Autodesk Fusion 360 part; units mm, degrees
(part 2 of 2)
sketch "Sketch1" plane through (0, 0, 0) normal (0, 0, 1) x (1, 0, 0) in component "Component"
  spline S0 degree 5 poles (13.995984, -1.682277) (13.996145, -1.682295) (13.99649, -1.682333) (13.997074, -1.682393) (13.997986, -1.682484) (13.999345, -1.682614) (14.000924, -1.682758) (14.002718, -1.682916) (14.004722, -1.683085) (14.006931, -1.683262) (14.009338, -1.683445) (14.011941, -1.683633) (14.014736, -1.683823) (14.01772, -1.684015) (14.020889, -1.684207) (14.024241, -1.684397) (14.027771, -1.684584) (14.031477, -1.684766) (14.035355, -1.684942) (14.039402, -1.685111) (14.043617, -1.685272) (14.047995, -1.685422) (14.052535, -1.685562) (14.057234, -1.685689) (14.062089, -1.685804) (14.067098, -1.685904) (14.072259, -1.685988) (14.077569, -1.686056) (14.083026, -1.686107) (14.088629, -1.68614) (14.094374, -1.686154) (14.100261, -1.686147) (14.106286, -1.686119) (14.112449, -1.68607) (14.118747, -1.685998) (14.125178, -1.685903) (14.13174, -1.685783) (14.138433, -1.685639) (14.145254, -1.685469) (14.152202, -1.685272) (14.159274, -1.685049) (14.16647, -1.684797) (14.173787, -1.684518) (14.181225, -1.684209) (14.188782, -1.68387) (14.196456, -1.683501) (14.204247, -1.683101) (14.212151, -1.68267) (14.220169, -1.682207) (14.228299, -1.681711) (14.23654, -1.681182) (14.24489, -1.680619) (14.253348, -1.680022) (14.261913, -1.67939) (14.270584, -1.678723) (14.279359, -1.67802) (14.288238, -1.677281) (14.297218, -1.676505) (14.3063, -1.675692) (14.315482, -1.674842) (14.324762, -1.673954) (14.334141, -1.673027) (14.343616, -1.672061) (14.353187, -1.671056) (14.362853, -1.670012) (14.372612, -1.668927) (14.382464, -1.667802) (14.392408, -1.666636) (14.402443, -1.665429) (14.412568, -1.66418) (14.422782, -1.66289) (14.433084, -1.661557) (14.443473, -1.660182) (14.453948, -1.658763) (14.464509, -1.657302) (14.475155, -1.655797) (14.485884, -1.654247) (14.496696, -1.652654) (14.50759, -1.651016) (14.518565, -1.649334) (14.529621, -1.647606) (14.540757, -1.645833) (14.551972, -1.644014) (14.563264, -1.642149) (14.574634, -1.640238) (14.586081, -1.638281) (14.597604, -1.636276) (14.609202, -1.634225) (14.620874, -1.632127) (14.63262, -1.629981) (14.644439, -1.627787) (14.65633, -1.625545) (14.668293, -1.623255) (14.680327, -1.620916) (14.692431, -1.618529) (14.704605, -1.616093) (14.716848, -1.613607) (14.729159, -1.611073) (14.741538, -1.608488) (14.753984, -1.605854) (14.766497, -1.60317) (14.779075, -1.600436) (14.791718, -1.597652) (14.804426, -1.594816) (14.817198, -1.59193) (14.830033, -1.588994) (14.842931, -1.586006) (14.855891, -1.582966) (14.868913, -1.579875) (14.881995, -1.576733) (14.895139, -1.573538) (14.908342, -1.570292) (14.921604, -1.566993) (14.934926, -1.563642) (14.948305, -1.560239) (14.961743, -1.556783) (14.975237, -1.553274) (14.988788, -1.549712) (15.002395, -1.546097) (15.016058, -1.542429) (15.029776, -1.538707) (15.043548, -1.534932) (15.057375, -1.531103) (15.071255, -1.52722) (15.085188, -1.523283) (15.099173, -1.519292) (15.113211, -1.515247) (15.1273, -1.511148) (15.14144, -1.506993) (15.155631, -1.502785) (15.169872, -1.498521) (15.184163, -1.494203) (15.198502, -1.48983) (15.212891, -1.485402) (15.227328, -1.480918) (15.241812, -1.476379) (15.256344, -1.471785) (15.270923, -1.467135) (15.285548, -1.46243) (15.30022, -1.457669) (15.314936, -1.452852) (15.329698, -1.447979) (15.344505, -1.44305) (15.359356, -1.438064) (15.374251, -1.433023) (15.389189, -1.427925) (15.40417, -1.422771) (15.419194, -1.41756) (15.43426, -1.412293) (15.449368, -1.406969) (15.464517, -1.401588) (15.479707, -1.39615) (15.494937, -1.390656) (15.510208, -1.385104) (15.525518, -1.379495) (15.540868, -1.373829) (15.556256, -1.368106) (15.571683, -1.362325) (15.587148, -1.356487) (15.602651, -1.350592) (15.618192, -1.344639) (15.633769, -1.338628) (15.649383, -1.33256) (15.665034, -1.326434) (15.68072, -1.32025) (15.696441, -1.314008) (15.712198, -1.307708) (15.72799, -1.301351) (15.743816, -1.294935) (15.759676, -1.288461) (15.77557, -1.281929) (15.791497, -1.275338) (15.807457, -1.26869) (15.823449, -1.261983) (15.839474, -1.255217) (15.855531, -1.248393) (15.871619, -1.241511) (15.887739, -1.23457) (15.903889, -1.22757) (15.92007, -1.220512) (15.936281, -1.213395) (15.952522, -1.206219) (15.968793, -1.198985) (15.985093, -1.191692) (16.001421, -1.184339) (16.017778, -1.176928) (16.034164, -1.169458) (16.050577, -1.161929) (16.067018, -1.154341) (16.083486, -1.146694) (16.09998, -1.138988) (16.116502, -1.131222) (16.13305, -1.123398) (16.149623, -1.115514) (16.166222, -1.107571) (16.182847, -1.099569) (16.199497, -1.091508) (16.216171, -1.083387) (16.232869, -1.075206) (16.249592, -1.066967) (16.266339, -1.058668) (16.283109, -1.05031) (16.299902, -1.041892) (16.316718, -1.033414) (16.333556, -1.024878) (16.350417, -1.016281) (16.3673, -1.007625) (16.384205, -0.99891) (16.401131, -0.990135) (16.418077, -0.9813) (16.435045, -0.972406) (16.452034, -0.963452) (16.469042, -0.954438) (16.48607, -0.945365) (16.503119, -0.936232) (16.520186, -0.92704) (16.537273, -0.917787) (16.554378, -0.908475) (16.571502, -0.899104) (16.588644, -0.889672) (16.605804, -0.880181) (16.622982, -0.87063) (16.640177, -0.861019) (16.65739, -0.851349) (16.674619, -0.841618) (16.691864, -0.831828) (16.709127, -0.821978) (16.726405, -0.812068) (16.743699, -0.802099) (16.761008, -0.79207) (16.778333, -0.78198) (16.795673, -0.771831) (16.813028, -0.761623) (16.830397, -0.751354) (16.84778, -0.741025) (16.865177, -0.730637) (16.882588, -0.720189) (16.900012, -0.709681) (16.917449, -0.699113) (16.934898, -0.688486) (16.952361, -0.677798) (16.966342, -0.669201) (16.976834, -0.662726) (16.98383, -0.658397) (16.987329, -0.656229) knots 0 0 0 0 0 0 0.00416667 0.00833333 0.0125 0.01666667 0.02083333 0.025 0.02916667 0.03333333 0.0375 0.04166667 0.04583333 0.05 0.05416667 0.05833333 0.0625 0.06666667 0.07083333 0.075 0.07916667 0.08333333 0.0875 0.09166667 0.09583333 0.1 0.10416667 0.10833333 0.1125 0.11666667 0.12083333 0.125 0.12916667 0.13333333 0.1375 0.14166667 0.14583333 0.15 0.15416667 0.15833333 0.1625 0.16666667 0.17083333 0.175 0.17916667 0.18333333 0.1875 0.19166667 0.19583333 0.2 0.20416667 0.20833333 0.2125 0.21666667 0.22083333 0.225 0.22916667 0.23333333 0.2375 0.24166667 0.24583333 0.25 0.25416667 0.25833333 0.2625 0.26666667 0.27083333 0.275 0.27916667 0.28333333 0.2875 0.29166667 0.29583333 0.3 0.30416667 0.30833333 0.3125 0.31666667 0.32083333 0.325 0.32916667 0.33333333 0.3375 0.34166667 0.34583333 0.35 0.35416667 0.35833333 0.3625 0.36666667 0.37083333 0.375 0.37916667 0.38333333 0.3875 0.39166667 0.39583333 0.4 0.40416667 0.40833333 0.4125 0.41666667 0.42083333 0.425 0.42916667 0.43333333 0.4375 0.44166667 0.44583333 0.45 0.45416667 0.45833333 0.4625 0.46666667 0.47083333 0.475 0.47916667 0.48333333 0.4875 0.49166667 0.49583333 0.5 0.50416667 0.50833333 0.5125 0.51666667 0.52083333 0.525 0.52916667 0.53333333 0.5375 0.54166667 0.54583333 0.55 0.55416667 0.55833333 0.5625 0.56666667 0.57083333 0.575 0.57916667 0.58333333 0.5875 0.59166667 0.59583333 0.6 0.60416667 0.60833333 0.6125 0.61666667 0.62083333 0.625 0.62916667 0.63333333 0.6375 0.64166667 0.64583333 0.65 0.65416667 0.65833333 0.6625 0.66666667 0.67083333 0.675 0.67916667 0.68333333 0.6875 0.69166667 0.69583333 0.7 0.70416667 0.70833333 0.7125 0.71666667 0.72083333 0.725 0.72916667 0.73333333 0.7375 0.74166667 0.74583333 0.75 0.75416667 0.75833333 0.7625 0.76666667 0.77083333 0.775 0.77916667 0.78333333 0.7875 0.79166667 0.79583333 0.8 0.80416667 0.80833333 0.8125 0.81666667 0.82083333 0.825 0.82916667 0.83333333 0.8375 0.84166667 0.84583333 0.85 0.85416667 0.85833333 0.8625 0.86666667 0.87083333 0.875 0.87916667 0.88333333 0.8875 0.89166667 0.89583333 0.9 0.90416667 0.90833333 0.9125 0.91666667 0.92083333 0.925 0.92916667 0.93333333 0.9375 0.94166667 0.94583333 0.95 0.95416667 0.95833333 0.9625 0.96666667 0.97083333 0.975 0.97916667 0.98333333 0.9875 0.99166667 0.99583333 1 1 1 1 1 1
  spline S1 degree 5 poles (13.995984, 1.682277) (13.996145, 1.682295) (13.99649, 1.682333) (13.997074, 1.682393) (13.997986, 1.682484) (13.999345, 1.682614) (14.000924, 1.682758) (14.002718, 1.682916) (14.004722, 1.683085) (14.006931, 1.683262) (14.009338, 1.683445) (14.011941, 1.683633) (14.014736, 1.683823) (14.01772, 1.684015) (14.020889, 1.684207) (14.024241, 1.684397) (14.027771, 1.684584) (14.031477, 1.684766) (14.035355, 1.684942) (14.039402, 1.685111) (14.043617, 1.685272) (14.047995, 1.685422) (14.052535, 1.685562) (14.057234, 1.685689) (14.062089, 1.685804) (14.067098, 1.685904) (14.072259, 1.685988) (14.077569, 1.686056) (14.083026, 1.686107) (14.088629, 1.68614) (14.094374, 1.686154) (14.100261, 1.686147) (14.106286, 1.686119) (14.112449, 1.68607) (14.118747, 1.685998) (14.125178, 1.685903) (14.13174, 1.685783) (14.138433, 1.685639) (14.145254, 1.685469) (14.152202, 1.685272) (14.159274, 1.685049) (14.16647, 1.684797) (14.173787, 1.684518) (14.181225, 1.684209) (14.188782, 1.68387) (14.196456, 1.683501) (14.204247, 1.683101) (14.212151, 1.68267) (14.220169, 1.682207) (14.228299, 1.681711) (14.23654, 1.681182) (14.24489, 1.680619) (14.253348, 1.680022) (14.261913, 1.67939) (14.270584, 1.678723) (14.279359, 1.67802) (14.288238, 1.677281) (14.297218, 1.676505) (14.3063, 1.675692) (14.315482, 1.674842) (14.324762, 1.673954) (14.334141, 1.673027) (14.343616, 1.672061) (14.353187, 1.671056) (14.362853, 1.670012) (14.372612, 1.668927) (14.382464, 1.667802) (14.392408, 1.666636) (14.402443, 1.665429) (14.412568, 1.66418) (14.422782, 1.66289) (14.433084, 1.661557) (14.443473, 1.660182) (14.453948, 1.658763) (14.464509, 1.657302) (14.475155, 1.655797) (14.485884, 1.654247) (14.496696, 1.652654) (14.50759, 1.651016) (14.518565, 1.649334) (14.529621, 1.647606) (14.540757, 1.645833) (14.551972, 1.644014) (14.563264, 1.642149) (14.574634, 1.640238) (14.586081, 1.638281) (14.597604, 1.636276) (14.609202, 1.634225) (14.620874, 1.632127) (14.63262, 1.629981) (14.644439, 1.627787) (14.65633, 1.625545) (14.668293, 1.623255) (14.680327, 1.620916) (14.692431, 1.618529) (14.704605, 1.616093) (14.716848, 1.613607) (14.729159, 1.611073) (14.741538, 1.608488) (14.753984, 1.605854) (14.766497, 1.60317) (14.779075, 1.600436) (14.791718, 1.597652) (14.804426, 1.594816) (14.817198, 1.59193) (14.830033, 1.588994) (14.842931, 1.586006) (14.855891, 1.582966) (14.868913, 1.579875) (14.881995, 1.576733) (14.895139, 1.573538) (14.908342, 1.570292) (14.921604, 1.566993) (14.934926, 1.563642) (14.948305, 1.560239) (14.961743, 1.556783) (14.975237, 1.553274) (14.988788, 1.549712) (15.002395, 1.546097) (15.016058, 1.542429) (15.029776, 1.538707) (15.043548, 1.534932) (15.057375, 1.531103) (15.071255, 1.52722) (15.085188, 1.523283) (15.099173, 1.519292) (15.113211, 1.515247) (15.1273, 1.511148) (15.14144, 1.506993) (15.155631, 1.502785) (15.169872, 1.498521) (15.184163, 1.494203) (15.198502, 1.48983) (15.212891, 1.485402) (15.227328, 1.480918) (15.241812, 1.476379) (15.256344, 1.471785) (15.270923, 1.467135) (15.285548, 1.46243) (15.30022, 1.457669) (15.314936, 1.452852) (15.329698, 1.447979) (15.344505, 1.44305) (15.359356, 1.438064) (15.374251, 1.433023) (15.389189, 1.427925) (15.40417, 1.422771) (15.419194, 1.41756) (15.43426, 1.412293) (15.449368, 1.406969) (15.464517, 1.401588) (15.479707, 1.39615) (15.494937, 1.390656) (15.510208, 1.385104) (15.525518, 1.379495) (15.540868, 1.373829) (15.556256, 1.368106) (15.571683, 1.362325) (15.587148, 1.356487) (15.602651, 1.350592) (15.618192, 1.344639) (15.633769, 1.338628) (15.649383, 1.33256) (15.665034, 1.326434) (15.68072, 1.32025) (15.696441, 1.314008) (15.712198, 1.307708) (15.72799, 1.301351) (15.743816, 1.294935) (15.759676, 1.288461) (15.77557, 1.281929) (15.791497, 1.275338) (15.807457, 1.26869) (15.823449, 1.261983) (15.839474, 1.255217) (15.855531, 1.248393) (15.871619, 1.241511) (15.887739, 1.23457) (15.903889, 1.22757) (15.92007, 1.220512) (15.936281, 1.213395) (15.952522, 1.206219) (15.968793, 1.198985) (15.985093, 1.191692) (16.001421, 1.184339) (16.017778, 1.176928) (16.034164, 1.169458) (16.050577, 1.161929) (16.067018, 1.154341) (16.083486, 1.146694) (16.09998, 1.138988) (16.116502, 1.131222) (16.13305, 1.123398) (16.149623, 1.115514) (16.166222, 1.107571) (16.182847, 1.099569) (16.199497, 1.091508) (16.216171, 1.083387) (16.232869, 1.075206) (16.249592, 1.066967) (16.266339, 1.058668) (16.283109, 1.05031) (16.299902, 1.041892) (16.316718, 1.033414) (16.333556, 1.024878) (16.350417, 1.016281) (16.3673, 1.007625) (16.384205, 0.99891) (16.401131, 0.990135) (16.418077, 0.9813) (16.435045, 0.972406) (16.452034, 0.963452) (16.469042, 0.954438) (16.48607, 0.945365) (16.503119, 0.936232) (16.520186, 0.92704) (16.537273, 0.917787) (16.554378, 0.908475) (16.571502, 0.899104) (16.588644, 0.889672) (16.605804, 0.880181) (16.622982, 0.87063) (16.640177, 0.861019) (16.65739, 0.851349) (16.674619, 0.841618) (16.691864, 0.831828) (16.709127, 0.821978) (16.726405, 0.812068) (16.743699, 0.802099) (16.761008, 0.79207) (16.778333, 0.78198) (16.795673, 0.771831) (16.813028, 0.761623) (16.830397, 0.751354) (16.84778, 0.741025) (16.865177, 0.730637) (16.882588, 0.720189) (16.900012, 0.709681) (16.917449, 0.699113) (16.934898, 0.688486) (16.952361, 0.677798) (16.966342, 0.669201) (16.976834, 0.662726) (16.98383, 0.658397) (16.987329, 0.656229) knots 0 0 0 0 0 0 0.00416667 0.00833333 0.0125 0.01666667 0.02083333 0.025 0.02916667 0.03333333 0.0375 0.04166667 0.04583333 0.05 0.05416667 0.05833333 0.0625 0.06666667 0.07083333 0.075 0.07916667 0.08333333 0.0875 0.09166667 0.09583333 0.1 0.10416667 0.10833333 0.1125 0.11666667 0.12083333 0.125 0.12916667 0.13333333 0.1375 0.14166667 0.14583333 0.15 0.15416667 0.15833333 0.1625 0.16666667 0.17083333 0.175 0.17916667 0.18333333 0.1875 0.19166667 0.19583333 0.2 0.20416667 0.20833333 0.2125 0.21666667 0.22083333 0.225 0.22916667 0.23333333 0.2375 0.24166667 0.24583333 0.25 0.25416667 0.25833333 0.2625 0.26666667 0.27083333 0.275 0.27916667 0.28333333 0.2875 0.29166667 0.29583333 0.3 0.30416667 0.30833333 0.3125 0.31666667 0.32083333 0.325 0.32916667 0.33333333 0.3375 0.34166667 0.34583333 0.35 0.35416667 0.35833333 0.3625 0.36666667 0.37083333 0.375 0.37916667 0.38333333 0.3875 0.39166667 0.39583333 0.4 0.40416667 0.40833333 0.4125 0.41666667 0.42083333 0.425 0.42916667 0.43333333 0.4375 0.44166667 0.44583333 0.45 0.45416667 0.45833333 0.4625 0.46666667 0.47083333 0.475 0.47916667 0.48333333 0.4875 0.49166667 0.49583333 0.5 0.50416667 0.50833333 0.5125 0.51666667 0.52083333 0.525 0.52916667 0.53333333 0.5375 0.54166667 0.54583333 0.55 0.55416667 0.55833333 0.5625 0.56666667 0.57083333 0.575 0.57916667 0.58333333 0.5875 0.59166667 0.59583333 0.6 0.60416667 0.60833333 0.6125 0.61666667 0.62083333 0.625 0.62916667 0.63333333 0.6375 0.64166667 0.64583333 0.65 0.65416667 0.65833333 0.6625 0.66666667 0.67083333 0.675 0.67916667 0.68333333 0.6875 0.69166667 0.69583333 0.7 0.70416667 0.70833333 0.7125 0.71666667 0.72083333 0.725 0.72916667 0.73333333 0.7375 0.74166667 0.74583333 0.75 0.75416667 0.75833333 0.7625 0.76666667 0.77083333 0.775 0.77916667 0.78333333 0.7875 0.79166667 0.79583333 0.8 0.80416667 0.80833333 0.8125 0.81666667 0.82083333 0.825 0.82916667 0.83333333 0.8375 0.84166667 0.84583333 0.85 0.85416667 0.85833333 0.8625 0.86666667 0.87083333 0.875 0.87916667 0.88333333 0.8875 0.89166667 0.89583333 0.9 0.90416667 0.90833333 0.9125 0.91666667 0.92083333 0.925 0.92916667 0.93333333 0.9375 0.94166667 0.94583333 0.95 0.95416667 0.95833333 0.9625 0.96666667 0.97083333 0.975 0.97916667 0.98333333 0.9875 0.99166667 0.99583333 1 1 1 1 1 1
  spline S2 degree 5 poles (13.994657, -1.68213) (13.994711, -1.682136) (13.994817, -1.682148) (13.994976, -1.682166) (13.995188, -1.682189) (13.995453, -1.682218) (13.995665, -1.682242) (13.995825, -1.68226) (13.995931, -1.682271) (13.995984, -1.682277) knots 0 0 0 0 0 0 0.2 0.4 0.6 0.8 1 1 1 1 1 1
  spline S3 degree 5 poles (13.994657, 1.68213) (13.994711, 1.682136) (13.994817, 1.682148) (13.994976, 1.682166) (13.995188, 1.682189) (13.995453, 1.682218) (13.995665, 1.682242) (13.995825, 1.68226) (13.995931, 1.682271) (13.995984, 1.682277) knots 0 0 0 0 0 0 0.2 0.4 0.6 0.8 1 1 1 1 1 1
  line L0 (0, 0) -> (13.994657, -1.68213)
  line L1 (0, 0) -> (13.994657, 1.68213)
  arc A0 (16.987329, -0.656229) -> (16.987329, 0.656229) centre (0, 0) ccw
  point P0 (13.999968, -1.68267)
  point P1 (14.006616, -1.683235)
  point P2 (14.015933, -1.683899)
  point P3 (14.027922, -1.684588)
  point P4 (14.042586, -1.68523)
  point P5 (14.059926, -1.68575)
  point P6 (14.079939, -1.686076)
  point P7 (14.102623, -1.686133)
  point P8 (14.127975, -1.685849)
  point P9 (14.155988, -1.68515)
  point P10 (14.186656, -1.683962)
  point P11 (14.21997, -1.682212)
  point P12 (14.255919, -1.679828)
  point P13 (14.294493, -1.676737)
  point P14 (14.335677, -1.672865)
  point P15 (14.379458, -1.668141)
  point P16 (14.425819, -1.662492)
  point P17 (14.474742, -1.655848)
  point P18 (14.526208, -1.648135)
  point P19 (14.580197, -1.639283)
  point P20 (14.636686, -1.629221)
  point P21 (14.695653, -1.617879)
  point P22 (14.757071, -1.605187)
  point P23 (14.820915, -1.591075)
  point P24 (14.887156, -1.575474)
  point P25 (14.955766, -1.558315)
  point P26 (15.026712, -1.539532)
  point P27 (15.099964, -1.519055)
  point P28 (15.175488, -1.496819)
  point P29 (15.253247, -1.472757)
  point P30 (15.333207, -1.446804)
  point P31 (15.415329, -1.418894)
  point P32 (15.499574, -1.388964)
  point P33 (15.585901, -1.356949)
  point P34 (15.674269, -1.322787)
  point P35 (15.764635, -1.286416)
  point P36 (15.856953, -1.247775)
  point P37 (15.951178, -1.206804)
  point P38 (16.047263, -1.163441)
  point P39 (16.14516, -1.11763)
  point P40 (16.244818, -1.069312)
  point P41 (16.346188, -1.01843)
  point P42 (16.449216, -0.964928)
  point P43 (16.553849, -0.908752)
  point P44 (16.660034, -0.849846)
  point P45 (16.767714, -0.788158)
  point P46 (16.876831, -0.723636)
  point P47 (13.999968, 1.68267)
  point P48 (14.006616, 1.683235)
  point P49 (14.015933, 1.683899)
  point P50 (14.027922, 1.684588)
  point P51 (14.042586, 1.68523)
  point P52 (14.059926, 1.68575)
  point P53 (14.079939, 1.686076)
  point P54 (14.102623, 1.686133)
  point P55 (14.127975, 1.685849)
  point P56 (14.155988, 1.68515)
  point P57 (14.186656, 1.683962)
  point P58 (14.21997, 1.682212)
  point P59 (14.255919, 1.679828)
  point P60 (14.294493, 1.676737)
  point P61 (14.335677, 1.672865)
  point P62 (14.379458, 1.668141)
  point P63 (14.425819, 1.662492)
  point P64 (14.474742, 1.655848)
  point P65 (14.526208, 1.648135)
  point P66 (14.580197, 1.639283)
  point P67 (14.636686, 1.629221)
  point P68 (14.695653, 1.617879)
  point P69 (14.757071, 1.605187)
  point P70 (14.820915, 1.591075)
  point P71 (14.887156, 1.575474)
  point P72 (14.955766, 1.558315)
  point P73 (15.026712, 1.539532)
  point P74 (15.099964, 1.519055)
  point P75 (15.175488, 1.496819)
  point P76 (15.253247, 1.472757)
  point P77 (15.333207, 1.446804)
  point P78 (15.415329, 1.418894)
  point P79 (15.499574, 1.388964)
  point P80 (15.585901, 1.356949)
  point P81 (15.674269, 1.322787)
  point P82 (15.764635, 1.286416)
  point P83 (15.856953, 1.247775)
  point P84 (15.951178, 1.206804)
  point P85 (16.047263, 1.163441)
  point P86 (16.14516, 1.11763)
  point P87 (16.244818, 1.069312)
  point P88 (16.346188, 1.01843)
  point P89 (16.449216, 0.964928)
  point P90 (16.553849, 0.908752)
  point P91 (16.660034, 0.849846)
  point P92 (16.767714, 0.788158)
  point P93 (16.876831, 0.723636)
sketch "Sketch2" plane through (0, 0, 0) normal (0, 0, 1) x (1, 0, 0) in component "Component"
  circle A0 centre (0, 0) radius 12.5
extrude "Extrude1" add sketch "Sketch2" along normal blind 6.35 contours A0 picked at (-3.387945, -0.621009) makes body 1 in component "Component"
extrude "Extrude2" add sketch "Sketch1" along normal blind 6.35 separate body contours S0 S1 L0 L1 A0 picked at (9.330656, 0) makes body 2 in component "Component"
pattern_circular "C-Pattern1" count 15 over 360 about axis through (0, 0, 1.75) along (0, 0, 1) of "Extrude2" makes body 3 at (4.49007, 1.385281, 2.116667) makes body 4 at (3.538439, 3.091793, 2.116667) makes body 5 at (0.908352, 4.610275, 2.116667) makes body 6 at (0.070028, 4.698386, 2.116667) makes body 7 at (-2.818296, 3.759913, 2.116667) makes body 8 at (-3.444724, 3.195875, 2.116667) makes body 9 at (-4.446791, 1.518481, 2.116667) makes body 10 at (-4.679968, -0.421471, 2.116667) makes body 11 at (-4.103935, -2.288547, 2.116667) makes body 12 at (-2.818296, -3.759913, 2.116667) makes body 13 at (0.070028, -4.698386, 2.116667) makes body 14 at (1.974979, -4.263706, 2.116667) makes body 15 at (3.538439, -3.091793, 2.116667) makes body 16 at (4.033908, -2.409839, 2.116667) in component "Component"
combine "Combine1" operation add target body 1 tool bodies 2 3 4 5 6 7 8 9 10 11 12 13 14 15 16 in component "Component"
sketch "Sketch3" plane through (0, 0, 0) normal (0, 0, 1) x (1, 0, 0) in component "Component"
  line L0 (0, 0) -> (50.859375, 0) construction
  line L1 (50.859375, 0) -> (50.859375, 3) construction
  line L2 (50.859375, 3) -> (0, 3) construction
  line L3 (0, 3) -> (0, 0) construction
  constraint perpendicular L0 L1
  constraint parallel L0 L2
  constraint parallel L1 L3
ref_plane "WorkPlane1" through (0.130063, 0, 6.35) normal (0, 0, 1) x (1, 0, 0)
sketch "Sketch1 (2)" plane through (0, 0, 6.35) normal (0, 0, 1) x (1, 0, 0)
  circle A0 centre (0, 0) radius 12.5
  circle A1 centre (0, 0) radius 20
  line L0 (0, 0) -> (-20, 0)
  line L1 (0, 0) -> (16.18034, -11.755705)
  point P0 (2.416381, 12.264221)
  dimension "d15" = 40
  dimension "d16" = 216
  constraint coincident A0.centre A1.centre
  constraint coincident A1 L0.end
  constraint horizontal L0
  measures "d15" diameter of A1
extrude "Extrude3" cut sketch "Sketch1 (2)" against normal through all contours A0 A1 L0 L1 picked at (13.124223, -11.507785) bodies 1 in component "Component"
component "Component" placed x (1, 0, 0) y (0, 1, 0) z (0, 0, 1) at (0, 0, 0)
equation "NumTeeth = 9"
equation "d16 = ( 24 * NumTeeth ) * 1 deg"

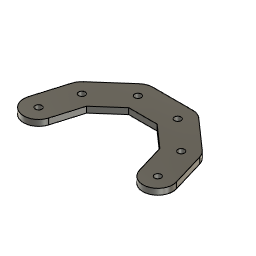
design "GearPlateV2"
Autodesk Fusion 360 part; units mm, degrees
sketch "Sketch1" plane through (0, 0, 0) normal (0, 0, 1) x (1, 0, 0)
  circle A0 centre (0, 0) radius 3.275
  circle A1 centre (120, 0) radius 3.275
  circle A2 centre (120, 0) radius 15 construction
  circle A3 centre (0, 0) radius 15 construction
  circle A4 centre (120, 0) radius 15 construction
  circle A5 centre (10, 33.541) radius 20 construction
  circle A6 centre (40, 59.9985) radius 20 construction
  circle A7 centre (110, 33.541) radius 20 construction
  circle A8 centre (80, 59.9985) radius 20 construction
  circle A9 centre (109.7709, 71.7327) radius 12 construction
  line L0 (143.6237, 88.934) -> (255.6237, 88.934) construction
  circle A10 centre (59.9233, -6.3144) radius 27.5 construction
  circle A11 centre (0, 0) radius 15 construction
  line L1 (150, 0) -> (-15, 0) construction
  circle A12 centre (0, 0) radius 17 construction
  circle A13 centre (120, 0) radius 17 construction
  circle A14 centre (10, 33.541) radius 3.275
  circle A15 centre (40, 59.9985) radius 3.275
  circle A16 centre (80, 59.9985) radius 3.275
  circle A17 centre (110, 33.541) radius 3.275
  circle A18 centre (0, 0) radius 15
  circle A19 centre (10, 33.541) radius 15
  circle A20 centre (40, 59.9985) radius 15
  circle A21 centre (80, 59.9985) radius 15
  circle A22 centre (110, 33.541) radius 15
  circle A23 centre (120, 0) radius 15
  line L2 (-14.3747, 4.2857) -> (-4.3747, 37.8267)
  line L3 (0.0784, 44.791) -> (30.0784, 71.2485)
  line L4 (40, 74.9985) -> (80, 74.9985)
  line L5 (14.3747, -4.2857) -> (24.3747, 29.2553)
  line L6 (19.9216, 22.291) -> (49.9216, 48.7485)
  line L7 (40, 44.9985) -> (80, 44.9985)
  line L8 (70.0784, 48.7485) -> (100.0784, 22.291)
  line L9 (89.9216, 71.2485) -> (119.9216, 44.791)
  line L10 (95.6253, 29.2553) -> (105.6253, -4.2857)
  line L11 (124.3747, 37.8267) -> (134.3747, 4.2857)
  point P0 (105, 0)
  point P1 (15, 0)
  dimension "d2" = 6.55
  dimension "d3" = 6.55
  dimension "d4" = 120
  dimension "d7" = 30
  dimension "d10" = 30
  dimension "d11" = 30
  dimension "d20" = 40
  dimension "d26" = 24
  dimension "d27" = 112
  dimension "d28" = 55
  dimension "d31" = 30
  dimension "d33" = 165
  dimension "d35" = 90
  dimension "d36" = 100
  dimension "d37" = 34
  dimension "d38" = 34
  dimension "d40" = 6.55
  dimension "d41" = 6.55
  dimension "d42" = 6.55
  dimension "d43" = 6.55
  dimension "d44" = 30
  dimension "d45" = 30
  dimension "d46" = 30
  dimension "d47" = 30
  dimension "d48" = 30
  dimension "d49" = 30
  constraint coincident A0.centre A3.centre
  constraint horizontal A0.centre A1.centre
  constraint concentric A1 A2
  constraint concentric A0 A3
  constraint concentric A1 A4
  constraint tangent A3 A5
  constraint tangent A4 A7
  constraint tangent A7 A8
  constraint tangent A6 A8
  constraint tangent A5 A6
  constraint tangent A8 A9
  constraint horizontal L0
  constraint horizontal A6.centre A8.centre
  constraint horizontal A5.centre A7.centre
  constraint concentric A3 A11
  constraint coincident A11 L1.end
  constraint horizontal L1
  constraint coincident A2 P0
  constraint coincident L1 P0
  constraint coincident A11 P1
  constraint coincident L1 P1
  constraint equal A5 A6
  constraint equal A6 A8
  constraint equal A7 A8
  constraint concentric A3 A12
  constraint concentric A4 A13
  constraint concentric A5 A14
  constraint concentric A6 A15
  constraint concentric A8 A16
  constraint concentric A7 A17
  constraint concentric A12 A18
  constraint concentric A14 A19
  constraint concentric A6 A20
  constraint concentric A16 A21
  constraint concentric A17 A22
  constraint concentric A1 A23
  constraint coincident A3 L2.start
  constraint coincident A19 L2.end
  constraint tangent A19 L2
  constraint coincident A19 L3.start
  constraint coincident A20 L3.end
  constraint tangent A20 L3
  constraint coincident A20 L4.start
  constraint coincident A21 L4.end
  constraint tangent A21 L4
  constraint coincident A3 L5.start
  constraint coincident A19 L5.end
  constraint tangent A19 L5
  constraint coincident A19 L6.start
  constraint coincident A20 L6.end
  constraint tangent A20 L6
  constraint coincident A20 L7.start
  constraint coincident A21 L7.end
  constraint tangent A21 L7
  constraint coincident A21 L8.start
  constraint coincident A22 L8.end
  constraint tangent A22 L8
  constraint coincident A21 L9.start
  constraint coincident A22 L9.end
  constraint tangent A22 L9
  constraint coincident A22 L10.start
  constraint coincident A2 L10.end
  constraint tangent A2 L10
  constraint coincident A22 L11.start
  constraint coincident A2 L11.end
  constraint tangent A2 L11
  constraint tangent A22 L11
  constraint tangent A22 L10
  constraint tangent A21 L8
  constraint tangent A21 L9
  constraint tangent A20 L4
  constraint tangent A20 L7
  constraint tangent A19 L6
  constraint tangent A3 L5
  constraint tangent A3 L2
  constraint tangent A19 L3
  measures "d2" diameter of A0
  measures "d3" diameter of A1
  measures "d4" distance of A0.centre A1.centre
  measures "d7" diameter of A2
  measures "d10" diameter of A3
  measures "d11" diameter of A4
  measures "d20" diameter of A5
  measures "d26" diameter of A9
  measures "d27" distance of L0.start L0.end
  measures "d28" diameter of A10
  measures "d31" diameter of A11
  measures "d33" distance of L1.start L1.end
  measures "d35" distance of P0 P1
  measures "d36" distance of A5.centre A7.centre
  measures "d37" diameter of A12
  measures "d38" diameter of A13
  measures "d40" diameter of A14
  measures "d41" diameter of A15
  measures "d42" diameter of A16
  measures "d43" diameter of A17
  measures "d44" diameter of A18
  measures "d45" diameter of A19
  measures "d46" diameter of A20
  measures "d47" diameter of A21
  measures "d48" diameter of A22
  measures "d49" diameter of A23
extrude "Extrude2" add sketch "Sketch1" along normal blind 6
equation "SlipGearNominal = 209.5 mm"
equation "d2 = HoleSize"
equation "d3 = HoleSize"
equation "SlipGearOffset = 0.5 mm"
equation "HoleSize = 6.55 mm"
equation "d40 = HoleSize"
equation "d41 = HoleSize"
equation "d42 = HoleSize"
equation "d43 = HoleSize"
